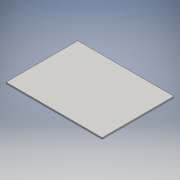
# Autodesk Inventor part: botn
Saved by Autodesk Inventor 2016 (Build 200138000, 138)
## iProperties
Created: 2016-02-20
Part Number: botn
Material: Generic
Document SubType Name: Modeling
Designer: Róbert
Density: 1 g/cm^3
Appearance: Default
Author: Róbert
Autodesk Inventor part; units mm, degrees
ref_plane "YZ Plane" through (0, 0, 0) normal (1, 0, 0) x (0, 1, 0)
ref_plane "XZ Plane" through (0, 0, 0) normal (0, 1, 0) x (-1, 0, 0)
ref_plane "XY Plane" through (0, 0, 0) normal (0, 0, 1) x (1, 0, 0)
sketch "Sketch1" plane through (0, 0, 0) normal (0, 0, 1) x (1, 0, 0)
  line L0 (0, 0) -> (0, 50)
  line L1 (0, 50) -> (-67, 50)
  line L2 (-67, 50) -> (-67, 0)
  line L3 (-67, 0) -> (0, 0)
  dimension "d0" = 50
  dimension "d1" = 67
  dimension "d2" = 50
  dimension "d3" = 67
  constraints: 8 end point, 2 perpendicular, 1 vertical
  measures "d0" distance of L0.start L0.end
  measures "d1" distance of L0.end L1.end
  measures "d2" distance of L1.end L2.end
  measures "d3" distance of L2.end L0.start
extrude "Extrusion1" add sketch "Sketch1" along normal blind 1
body "Solid1"
